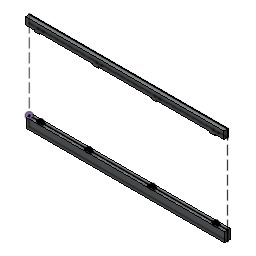
aspire keyboard tray v6 (Autodesk Fusion 360 design; units mm, degrees)
Autodesk Fusion 360 part; units mm, degrees
sketch "Sketch1" plane through (0, 0, 0) normal (0, 1, 0) x (1, 0, 0)
  line L0 (0, 0) -> (271.5, 0)
  line L1 (271.5, 0) -> (271.5, 3)
  line L2 (271.5, 3) -> (0, 3) construction
  line L3 (0, 3) -> (0, 0)
  line L4 (271.5, 3) -> (271.5, 13)
  line L5 (271.5, 13) -> (0, 13)
  line L6 (0, 13) -> (0, 3)
  line L7 (11.15, 0) -> (12.8821, 3)
  line L8 (77.3, 0) -> (79.0321, 3)
  line L9 (164.2, 0) -> (165.9321, 3)
  line L10 (251.2, 0) -> (252.9321, 3)
  line L11 (20.15, 0) -> (18.4179, 3)
  line L12 (84.5679, 3) -> (86.3, 0)
  line L13 (171.4679, 3) -> (173.2, 0)
  line L14 (258.4679, 3) -> (260.2, 0)
  line L15 (252.9321, 3) -> (258.4679, 3)
  line L16 (165.9321, 3) -> (171.4679, 3)
  line L17 (12.8821, 3) -> (18.4179, 3)
  line L18 (79.0321, 3) -> (84.5679, 3)
  line L19 (11.15, 0) -> (20.15, 0) construction
  line L20 (86.3, 0) -> (77.3, 0) construction
  line L21 (173.2, 0) -> (164.2, 0) construction
  line L22 (260.2, 0) -> (251.2, 0) construction
  line L23 (0, 0) -> (271.5, 0) construction
  line L24 (271.5, 0) -> (271.5, -110) construction
  line L25 (271.5, -110) -> (0, -110) construction
  line L26 (0, -110) -> (0, 0) construction
  line L27 (0, -108.5) -> (271.5, -108.5) construction
  line L28 (259.3, -110) -> (259.3, -108.5)
  line L29 (252, -110) -> (252, -108.5)
  line L30 (179.3, -110) -> (179.3, -108.5)
  line L31 (172, -110) -> (172, -108.5)
  line L32 (99.5, -110) -> (99.5, -108.5)
  line L33 (92.3, -110) -> (92.3, -108.5)
  line L34 (12, -110) -> (12, -108.5)
  line L35 (19.3, -110) -> (19.3, -108.5)
  line L36 (0, -110) -> (271.5, -110)
  line L37 (271.5, -110) -> (271.5, -120)
  line L38 (271.5, -120) -> (0, -120)
  line L39 (0, -120) -> (0, -110)
  line L40 (12, -108.5) -> (19.3, -108.5)
  line L41 (92.3, -108.5) -> (99.5, -108.5)
  line L42 (172, -108.5) -> (179.3, -108.5)
  line L43 (252, -108.5) -> (259.3, -108.5)
  point P0 (255.7, 0)
  point P1 (168.7, 0)
  point P2 (81.8, 0)
  point P3 (15.65, 0)
  dimension "d1" = 271.5
  dimension "d2" = 3
  dimension "d3" = 10
  dimension "d4" = 60
  dimension "d9" = 60
  dimension "d18" = 9
  dimension "d19" = 168.7
  dimension "d20" = 255.7
  dimension "d21" = 81.8
  dimension "d22" = 15.65
  dimension "d23" = 110
  dimension "d24" = 1.5
  dimension "d25" = 12.2
  dimension "d26" = 19.5
  dimension "d27" = 92.2
  dimension "d28" = 99.5
  dimension "d29" = 172
  dimension "d30" = 179.2
  dimension "d31" = 259.5
  dimension "d32" = 252.2
  dimension "d33" = 10
  constraint horizontal L0
  constraint vertical L1
  constraint horizontal L2
  constraint vertical L3
  constraint coincident L0.start L3.end
  constraint vertical L4
  constraint horizontal L5
  constraint vertical L6
  constraint coincident L1.end L2.start
  constraint coincident L0 L7.start
  constraint coincident L2 L7.end
  constraint coincident L0 L8.start
  constraint coincident L2 L8.end
  constraint parallel L7 L8
  constraint coincident L0 L9.start
  constraint coincident L2 L9.end
  constraint parallel L8 L9
  constraint coincident L0 L10.start
  constraint coincident L2 L10.end
  constraint parallel L9 L10
  constraint coincident L0 L11.start
  constraint coincident L2 L11.end
  constraint coincident L2 L12.start
  constraint coincident L0 L12.end
  constraint parallel L11 L12
  constraint coincident L2 L13.start
  constraint coincident L0 L13.end
  constraint parallel L12 L13
  constraint coincident L2 L14.start
  constraint coincident L0 L14.end
  constraint parallel L13 L14
  constraint equal L21 L22
  constraint midpoint L22 P0
  constraint midpoint L21 P1
  constraint midpoint L20 P2
  constraint midpoint L19 P3
  constraint equal L20 L21
  constraint equal L19 L20
  constraint horizontal L23
  constraint vertical L24
  constraint horizontal L25
  constraint vertical L26
  constraint coincident L0.end L1.start
  constraint coincident L26 L27.start
  constraint coincident L24 L27.end
  constraint perpendicular L24 L27
  constraint coincident L25 L28.start
  constraint coincident L27 L28.end
  constraint perpendicular L27 L28
  constraint coincident L25 L29.start
  constraint coincident L27 L29.end
  constraint perpendicular L27 L29
  constraint coincident L25 L30.start
  constraint coincident L27 L30.end
  constraint perpendicular L27 L30
  constraint coincident L25 L31.start
  constraint coincident L27 L31.end
  constraint perpendicular L27 L31
  constraint coincident L25 L32.start
  constraint coincident L27 L32.end
  constraint perpendicular L27 L32
  constraint coincident L25 L33.start
  constraint coincident L27 L33.end
  constraint perpendicular L27 L33
  constraint coincident L25 L34.start
  constraint coincident L27 L34.end
  constraint perpendicular L27 L34
  constraint coincident L25 L35.start
  constraint coincident L27 L35.end
  constraint perpendicular L27 L35
  constraint horizontal L36
  constraint vertical L37
  constraint horizontal L38
  constraint vertical L39
  constraint coincident L24.end L25.start
  measures "d1" distance of L0.start L0.end
  measures "d2" distance of L0.start L2.end
  measures "d3" distance of L2.end L5.end
  measures "d4" angle of L0 L7
  measures "d9" angle of L0 L11
  measures "d18" distance of L10.start L14.end
  measures "d19" distance of L0.start P1
  measures "d20" distance of L0.start P0
  measures "d21" distance of L0.start P2
  measures "d22" distance of L0.start P3
  measures "d23" distance of L0.end L24.end
  measures "d24" distance of L25.end L27.start
  measures "d25" distance of L24.end L28.start
  measures "d26" distance of L27.end L29.end
  measures "d27" distance of L24.end L30.start
  measures "d28" distance of L27.end L31.end
  measures "d29" distance of L24.end L32.start
  measures "d30" distance of L27.end L33.end
  measures "d31" distance of L27.end L34.end
  measures "d32" distance of L24.end L35.start
  measures "d33" distance of L25.end L38.end
extrude "Extrude1" add sketch "Sketch1" along normal mid plane 8 contours L0 L1 L3 L4 L5 L6 L7 L8 L9 L10 L11 L12 L13 L14 L15 L16 L17 L18 | L0 L7 L11 L17 | L0 L8 L12 L18 | L0 L9 L13 L16 | L0 L10 L14 L15 makes body 1
extrude "Extrude2" cut sketch "Sketch1" along normal mid plane 4 contours L0 L7 L11 L17 | L0 L8 L12 L18 | L0 L9 L13 L16 | L0 L10 L14 L15 bodies 1
extrude "Extrude3" add sketch "Sketch1" against normal blind 5 separate body contours L28 L29 L36 L43 | L36 L37 L38 L39 | L30 L31 L36 L42 | L32 L33 L36 L41 | L34 L35 L36 L40 makes body 2
extrude "Extrude4" add sketch "Sketch1" along normal blind 1 contours L36 L37 L38 L39 bodies 2
